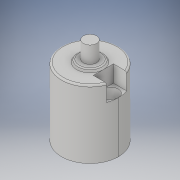
# Autodesk Inventor part: BaseEje
Saved by Autodesk Inventor 2019 (Build 230136000, 136)
## iProperties
Created: 2020-08-07
Part Number: BaseEje
Material: Generic
Document SubType Name: Modeling
Designer: Sergio
Density: 1 g/cm^3
Appearance: Default
Author: Sergio
Autodesk Inventor part; units mm, degrees
ref_plane "YZ Plane" through (0, 0, 0) normal (1, 0, 0) x (0, 1, 0)
ref_plane "XZ Plane" through (0, 0, 0) normal (0, 1, 0) x (-1, 0, 0)
ref_plane "XY Plane" through (0, 0, 0) normal (0, 0, 1) x (1, 0, 0)
sketch "Sketch1" plane through (0, 0, 0) normal (1, 0, 0) x (0, 1, 0)
  line L0 (0, 0) -> (52, 0)
  line L1 (52, 0) -> (52, -3.95)
  line L2 (52, -3.95) -> (42, -3.95)
  line L3 (42, -3.95) -> (42, -6.95)
  line L4 (42, -6.95) -> (40.5, -7.95)
  line L5 (0, -16.95) -> (0, 0)
  line L6 (-10.4, 0) -> (62.4, 0) projected
  line L7 (40.5, -7.95) -> (40.5, -16.95)
  line L8 (40.5, -16.95) -> (0, -16.95)
  dimension "d0" = 3.95
  dimension "d2" = 3
  dimension "d3" = 10
  dimension "d4" = 52
  dimension "d9" = 9
  dimension "d10" = 16.95
  dimension "d11" = 1.5
  constraints: 16 end point, 4 perpendicular, 1 horizontal, 1 vertical
  measures "d0" distance of L0.end L1.end
  measures "d2" distance of L2.end L3.end
  measures "d3" distance of L1.end L2.end
  measures "d4" distance of L0.start L0.end
  measures "d9" distance of L4.end L7.end
  measures "d10" distance of L5.start L0.start
  measures "d11" distance between parallel lines of L7 L3
revolve "Revolution1" add sketch "Sketch1" angle 360 about axis through (0, -10, 0) along (0, 1, 0)
sketch "Sketch2" plane through (0, 40.5, 0) normal (0, 1, 0) x (1, 0, 0)
  circle A0 centre (12.45, 0.0008) radius 4.5
  line L0 (16.95, 0.0008) -> (16.95, -33.7296) construction
  point P0 (0, 0)
  dimension "d12" = 9
  dimension "d13" = 4.5
  constraints: 2 end point, 1 horizontal alignment, 1 vertical, 2 other
  measures "d13" distance from line of L0 point (12.45, 0.001)
extrude "Extrusion1" cut sketch "Sketch2" against normal blind 50
sketch "Sketch4" plane through (12.45, 40.5, -0.0008) normal (0, 1, 0) x (1, 0, 0)
  line L0 (4.5, -6) -> (-4.5, -6)
  line L1 (-4.5, -6) -> (-4.5, 6)
  line L2 (-4.5, 6) -> (4.5, 6)
  line L3 (4.5, 6) -> (4.5, -6)
  line L4 (4.5, -6) -> (-4.5, 6) construction
  line L5 (-4.5, -6) -> (4.5, 6) construction
  point P0 (-12.45, -0.0004)
  point P1 (0, 0)
  dimension "d16" = 9
  dimension "d17" = 12
  constraints: 12 end point, 2 midpoint, 2 parallel, 1 horizontal, 1 perpendicular
  measures "d16" distance of L1.end L2.end
  measures "d17" distance of L0.end L1.end
extrude "Extrusion2" cut sketch "Sketch4" against normal blind 10
fillet "Fillet1" radius 1 3 edges at (0, 42, 6.95) (9.6329, 40.5, -13.9466) (-13.9461, 40.5, 9.6337)
body "Solid1"
